Autodesk Inventor part; units mm, degrees
(part 2 of 2)
sketch "Эскиз30" plane through (0, 0, 0) normal (-1, 0, 0) x (0, 0, 1)
  circle A0 centre (-371.0468, 185.0848) radius 1.625 projected
  circle A1 centre (-103, 60) radius 2.1 projected
  circle A2 centre (-135.25, 60) radius 2.1 projected
  circle A3 centre (-173.9908, 56.343) radius 2.1 projected
  circle A4 centre (-50.8872, 165.0002) radius 2.1 projected
  circle A5 centre (-287, 56.343) radius 2.1 projected
  circle A6 centre (-319.1128, 165.0002) radius 2.1 projected
  arc A7 (-250, 372) -> (-253, 375) centre (-253, 372) ccw projected
  line L0 (-253, 375) -> (-377, 375) projected
  arc A8 (-377, 375) -> (-380, 372) centre (-377, 372) ccw projected
  line L1 (-380, 372) -> (-380, -2) projected
  arc A9 (-380, -2) -> (-377, -5) centre (-377, -2) ccw projected
  line L2 (-377, -5) -> (7, -5) projected
  arc A10 (7, -5) -> (10, -2) centre (7, -2) ccw projected
  line L3 (10, -2) -> (10, 372) projected
  arc A11 (10, 372) -> (7, 375) centre (7, 372) ccw projected
  line L4 (7, 375) -> (-117, 375) projected
  arc A12 (-117, 375) -> (-120, 372) centre (-117, 372) ccw projected
  line L5 (-120, 372) -> (-120, 323.5966) projected
  arc A13 (-123, 320.5966) -> (-120, 323.5966) centre (-123, 323.5966) ccw projected
  line L6 (-123, 320.5966) -> (-247, 320.5966) projected
  arc A14 (-250, 323.5966) -> (-247, 320.5966) centre (-247, 323.5966) ccw projected
  line L7 (-250, 323.5966) -> (-250, 372) projected
  arc A15 (-43, 338.848) -> (-40, 341.848) centre (-43, 341.848) ccw projected
  line L8 (-40, 341.848) -> (-40, 367) projected
  arc A16 (-37, 370) -> (-40, 367) centre (-37, 367) ccw projected
  line L9 (-37, 370) -> (-1, 370) projected
  arc A17 (2, 367) -> (-1, 370) centre (-1, 367) ccw projected
  line L10 (2, 367) -> (2, 269.848) projected
  arc A18 (-1, 266.848) -> (2, 269.848) centre (-1, 269.848) ccw projected
  line L11 (-1, 266.848) -> (-49, 266.848) projected
  arc A19 (-52, 269.848) -> (-49, 266.848) centre (-49, 269.848) ccw projected
  line L12 (-52, 269.848) -> (-52, 335.848) projected
  arc A20 (-49, 338.848) -> (-52, 335.848) centre (-49, 335.848) ccw projected
  line L13 (-49, 338.848) -> (-43, 338.848) projected
  arc A21 (-40, 28.152) -> (-43, 31.152) centre (-43, 28.152) ccw projected
  line L14 (-43, 31.152) -> (-49, 31.152) projected
  arc A22 (-52, 34.152) -> (-49, 31.152) centre (-49, 34.152) ccw projected
  line L15 (-52, 34.152) -> (-52, 100.152) projected
  arc A23 (-49, 103.152) -> (-52, 100.152) centre (-49, 100.152) ccw projected
  line L16 (-49, 103.152) -> (-43, 103.152) projected
  arc A24 (-43, 103.152) -> (-40, 106.152) centre (-43, 106.152) ccw projected
  line L17 (-40, 106.152) -> (-40, 160) projected
  arc A25 (-37, 163) -> (-40, 160) centre (-37, 160) ccw projected
  line L18 (-37, 163) -> (-1, 163) projected
  arc A26 (2, 160) -> (-1, 163) centre (-1, 160) ccw projected
  line L19 (2, 160) -> (2, 3) projected
  arc A27 (-1, 0) -> (2, 3) centre (-1, 3) ccw projected
  line L20 (-1, 0) -> (-37, 0) projected
  arc A28 (-40, 3) -> (-37, 0) centre (-37, 3) ccw projected
  line L21 (-40, 3) -> (-40, 28.152) projected
  line L22 (-165, 8) -> (-165, 44) projected
  arc A29 (-162, 47) -> (-165, 44) centre (-162, 44) ccw projected
  line L23 (-162, 47) -> (-96, 47) projected
  arc A30 (-93, 44) -> (-96, 47) centre (-96, 44) ccw projected
  line L24 (-93, 44) -> (-93, 8) projected
  arc A31 (-96, 5) -> (-93, 8) centre (-96, 8) ccw projected
  line L25 (-96, 5) -> (-162, 5) projected
  arc A32 (-165, 8) -> (-162, 5) centre (-162, 8) ccw projected
  circle A33 centre (-152.75, 251.9941) radius 2.1 projected
  circle A34 centre (-217.25, 118.0059) radius 2.1 projected
  circle A35 centre (-217.25, 57.0059) radius 2.1 projected
  circle A36 centre (-217.25, 251.9941) radius 2.1 projected
  circle A37 centre (-152.75, 312.9941) radius 2.1 projected
  circle A38 centre (-152.75, 118.0059) radius 2.1 projected
  circle A39 centre (-152.75, 57.0059) radius 2.1 projected
  circle A40 centre (-217.25, 312.9941) radius 2.1 projected
  circle A41 centre (-124.375, 193.0059) radius 2 projected
  circle A42 centre (-124.375, 129.0059) radius 2 projected
  line L26 (-98.825, 137.3849) -> (-98.825, 226.3849) projected
  arc A43 (-95.825, 229.3849) -> (-98.825, 226.3849) centre (-95.825, 226.3849) ccw projected
  line L27 (-95.825, 229.3849) -> (-87.825, 229.3849) projected
  arc A44 (-84.825, 226.3849) -> (-87.825, 229.3849) centre (-87.825, 226.3849) ccw projected
  line L28 (-84.825, 226.3849) -> (-84.825, 137.3849) projected
  arc A45 (-87.825, 134.3849) -> (-84.825, 137.3849) centre (-87.825, 137.3849) ccw projected
  line L29 (-87.825, 134.3849) -> (-95.825, 134.3849) projected
  arc A46 (-98.825, 137.3849) -> (-95.825, 134.3849) centre (-95.825, 137.3849) ccw projected
  line L30 (-358.5, 185.5001) -> (-358.5, 244.5001) projected
  arc A47 (-355.5, 247.5001) -> (-358.5, 244.5001) centre (-355.5, 244.5001) ccw projected
  line L31 (-355.5, 247.5001) -> (-335, 247.5001) projected
  arc A48 (-332, 244.5001) -> (-335, 247.5001) centre (-335, 244.5001) ccw projected
  line L32 (-332, 244.5001) -> (-332, 185.5001) projected
  arc A49 (-335, 182.5001) -> (-332, 185.5001) centre (-335, 185.5001) ccw projected
  line L33 (-335, 182.5001) -> (-355.5, 182.5001) projected
  arc A50 (-358.5, 185.5001) -> (-355.5, 182.5001) centre (-355.5, 185.5001) ccw projected
  line L34 (-35, 247.5001) -> (-14.5, 247.5001) projected
  arc A51 (-11.5, 244.5001) -> (-14.5, 247.5001) centre (-14.5, 244.5001) ccw projected
  line L35 (-11.5, 244.5001) -> (-11.5, 185.5001) projected
  arc A52 (-14.5, 182.5001) -> (-11.5, 185.5001) centre (-14.5, 185.5001) ccw projected
  line L36 (-14.5, 182.5001) -> (-35, 182.5001) projected
  arc A53 (-38, 185.5001) -> (-35, 182.5001) centre (-35, 185.5001) ccw projected
  line L37 (-38, 185.5001) -> (-38, 244.5001) projected
  arc A54 (-35, 247.5001) -> (-38, 244.5001) centre (-35, 244.5001) ccw projected
  arc A55 (-185, 192.7028) -> (-185, 193.309) centre (-183.175, 193.0059) ccw projected
  line L38 (-185, 192.7028) -> (-185, 193.309) projected
  circle A56 centre (-376, 368.9) radius 2.1 projected
  circle A57 centre (-299, 142) radius 1.625 projected
  circle A58 centre (-299, 2.0002) radius 1.625 projected
  circle A59 centre (-54, 368) radius 1.625 projected
  circle A60 centre (6, 1.1) radius 2.1 projected
  circle A61 centre (6, 368.9) radius 2.1 projected
  circle A62 centre (-54, 142) radius 1.625 projected
  circle A63 centre (1, 228) radius 1.625 projected
  circle A64 centre (-316, 2.0002) radius 1.625 projected
  circle A65 centre (-371, 228) radius 1.625 projected
  circle A66 centre (-299, 368) radius 1.625 projected
  circle A67 centre (-183.175, 129.0059) radius 1.85 projected
  circle A68 centre (-316, 228) radius 1.625 projected
  circle A69 centre (-316, 142) radius 1.625 projected
  circle A70 centre (-71, 228) radius 1.625 projected
  circle A71 centre (-71, 368) radius 1.625 projected
  circle A72 centre (-54, 2.0002) radius 1.625 projected
  circle A73 centre (-71, 2.0002) radius 1.625 projected
  circle A74 centre (-71, 142) radius 1.625 projected
  circle A75 centre (-54, 228) radius 1.625 projected
  circle A76 centre (-376, 1.1) radius 2.1 projected
  circle A77 centre (-299, 228) radius 1.625 projected
  circle A78 centre (-316, 368) radius 1.625 projected
  arc A79 (-330, 341.848) -> (-327, 338.848) centre (-327, 341.848) ccw projected
  line L39 (-327, 338.848) -> (-321, 338.848) projected
  arc A80 (-318, 335.848) -> (-321, 338.848) centre (-321, 335.848) ccw projected
  line L40 (-318, 335.848) -> (-318, 269.848) projected
  arc A81 (-321, 266.848) -> (-318, 269.848) centre (-321, 269.848) ccw projected
  line L41 (-321, 266.848) -> (-369, 266.848) projected
  arc A82 (-372, 269.848) -> (-369, 266.848) centre (-369, 269.848) ccw projected
  line L42 (-372, 269.848) -> (-372, 367) projected
  arc A83 (-369, 370) -> (-372, 367) centre (-369, 367) ccw projected
  line L43 (-369, 370) -> (-333, 370) projected
  arc A84 (-330, 367) -> (-333, 370) centre (-333, 367) ccw projected
  line L44 (-330, 367) -> (-330, 341.848) projected
  arc A85 (-327, 31.152) -> (-330, 28.152) centre (-327, 28.152) ccw projected
  line L45 (-330, 28.152) -> (-330, 3) projected
  arc A86 (-333, 0) -> (-330, 3) centre (-333, 3) ccw projected
  line L46 (-333, 0) -> (-369, 0) projected
  arc A87 (-372, 3) -> (-369, 0) centre (-369, 3) ccw projected
  line L47 (-372, 3) -> (-372, 160) projected
  arc A88 (-369, 163) -> (-372, 160) centre (-369, 160) ccw projected
  line L48 (-369, 163) -> (-333, 163) projected
  arc A89 (-330, 160) -> (-333, 163) centre (-333, 160) ccw projected
  line L49 (-330, 160) -> (-330, 106.152) projected
  arc A90 (-330, 106.152) -> (-327, 103.152) centre (-327, 106.152) ccw projected
  line L50 (-327, 103.152) -> (-321, 103.152) projected
  arc A91 (-318, 100.152) -> (-321, 103.152) centre (-321, 100.152) ccw projected
  line L51 (-318, 100.152) -> (-318, 34.152) projected
  arc A92 (-321, 31.152) -> (-318, 34.152) centre (-321, 34.152) ccw projected
  line L52 (-321, 31.152) -> (-327, 31.152) projected
  line L53 (-224.75, 65.0059) -> (-224.75, 110.0059) projected
  line L54 (-282, 51.343) -> (-282, 61.343) projected
  line L55 (-268.3252, 69.343) -> (-228.25, 69.343)
  line L56 (-226.25, 71.343) -> (-226.25, 99.9959)
  line L57 (-235.9248, 106.343) -> (-276, 106.343)
  line L58 (-278, 104.343) -> (-278, 75.6902)
  line L59 (-278, 69.343) -> (-226.25, 106.343)
  line L60 (-269.4885, 72.97) -> (-229.4132, 101.6228)
  line L61 (-274.8368, 74.0633) -> (-234.7615, 102.7161)
  arc A93 (-269.4885, 72.97) -> (-268.3252, 69.343) centre (-268.3252, 71.343) ccw
  arc A94 (-278, 75.6902) -> (-274.8368, 74.0633) centre (-276, 75.6902) ccw
  arc A95 (-234.7615, 102.7161) -> (-235.9248, 106.343) centre (-235.9248, 104.343) ccw
  arc A96 (-276, 106.343) -> (-278, 104.343) centre (-276, 104.343) ccw
  arc A97 (-228.25, 69.343) -> (-226.25, 71.343) centre (-228.25, 71.343) ccw
  arc A98 (-226.25, 99.9959) -> (-229.4132, 101.6228) centre (-228.25, 99.9959) ccw
  line L62 (-185, -235.3635) -> (-185, 601.2713)
  line L63 (-101.6748, 69.343) -> (-141.75, 69.343)
  line L64 (-143.75, 71.343) -> (-143.75, 99.9959)
  line L65 (-134.0752, 106.343) -> (-94, 106.343)
  line L66 (-92, 104.343) -> (-92, 75.6902)
  line L67 (-92, 69.343) -> (-143.75, 106.343)
  line L68 (-100.5115, 72.97) -> (-140.5868, 101.6228)
  line L69 (-95.1632, 74.0633) -> (-135.2385, 102.7161)
  arc A99 (-101.6748, 69.343) -> (-100.5115, 72.97) centre (-101.6748, 71.343) ccw
  arc A100 (-95.1632, 74.0633) -> (-92, 75.6902) centre (-94, 75.6902) ccw
  arc A101 (-134.0752, 106.343) -> (-135.2385, 102.7161) centre (-134.0752, 104.343) ccw
  arc A102 (-92, 104.343) -> (-94, 106.343) centre (-94, 104.343) ccw
  arc A103 (-143.75, 71.343) -> (-141.75, 69.343) centre (-141.75, 71.343) ccw
  arc A104 (-140.5868, 101.6228) -> (-143.75, 99.9959) centre (-141.75, 99.9959) ccw
  line L70 (-268.3252, 133.343) -> (-228.25, 133.343)
  line L71 (-226.25, 135.343) -> (-226.25, 163.9959)
  line L72 (-235.9248, 170.343) -> (-276, 170.343)
  line L73 (-278, 168.343) -> (-278, 139.6902)
  line L74 (-278, 133.343) -> (-226.25, 170.343)
  line L75 (-269.4885, 136.97) -> (-229.4132, 165.6228)
  line L76 (-274.8368, 138.0633) -> (-234.7615, 166.7161)
  arc A105 (-269.4885, 136.97) -> (-268.3252, 133.343) centre (-268.3252, 135.343) ccw
  arc A106 (-278, 139.6902) -> (-274.8368, 138.0633) centre (-276, 139.6902) ccw
  arc A107 (-234.7615, 166.7161) -> (-235.9248, 170.343) centre (-235.9248, 168.343) ccw
  arc A108 (-276, 170.343) -> (-278, 168.343) centre (-276, 168.343) ccw
  arc A109 (-228.25, 133.343) -> (-226.25, 135.343) centre (-228.25, 135.343) ccw
  arc A110 (-226.25, 163.9959) -> (-229.4132, 165.6228) centre (-228.25, 163.9959) ccw
  line L77 (-458.8698, 185) -> (88.8698, 185) projected
  line L78 (-268.3252, 300.657) -> (-228.25, 300.657)
  line L79 (-226.25, 298.657) -> (-226.25, 270.0041)
  line L80 (-235.9248, 263.657) -> (-276, 263.657)
  line L81 (-278, 265.657) -> (-278, 294.3098)
  line L82 (-278, 300.657) -> (-226.25, 263.657)
  line L83 (-269.4885, 297.03) -> (-229.4132, 268.3772)
  line L84 (-274.8368, 295.9367) -> (-234.7615, 267.2839)
  arc A111 (-268.3252, 300.657) -> (-269.4885, 297.03) centre (-268.3252, 298.657) ccw
  arc A112 (-274.8368, 295.9367) -> (-278, 294.3098) centre (-276, 294.3098) ccw
  arc A113 (-235.9248, 263.657) -> (-234.7615, 267.2839) centre (-235.9248, 265.657) ccw
  arc A114 (-278, 265.657) -> (-276, 263.657) centre (-276, 265.657) ccw
  arc A115 (-226.25, 298.657) -> (-228.25, 300.657) centre (-228.25, 298.657) ccw
  arc A116 (-229.4132, 268.3772) -> (-226.25, 270.0041) centre (-228.25, 270.0041) ccw
  line L85 (-134.0752, 263.657) -> (-94, 263.657)
  arc A117 (-94, 263.657) -> (-92, 265.657) centre (-94, 265.657) ccw
  arc A118 (-135.2385, 267.2839) -> (-134.0752, 263.657) centre (-134.0752, 265.657) ccw
  arc A119 (-143.75, 270.0041) -> (-140.5868, 268.3772) centre (-141.75, 270.0041) ccw
  line L86 (-92, 265.657) -> (-92, 294.3098)
  line L87 (-95.1632, 295.9367) -> (-135.2385, 267.2839)
  line L88 (-92, 300.657) -> (-143.75, 263.657)
  arc A120 (-100.5115, 297.03) -> (-101.6748, 300.657) centre (-101.6748, 298.657) ccw
  arc A121 (-92, 294.3098) -> (-95.1632, 295.9367) centre (-94, 294.3098) ccw
  line L89 (-101.6748, 300.657) -> (-141.75, 300.657)
  line L90 (-143.75, 298.657) -> (-143.75, 270.0041)
  arc A122 (-141.75, 300.657) -> (-143.75, 298.657) centre (-141.75, 298.657) ccw
  line L91 (-100.5115, 297.03) -> (-140.5868, 268.3772)
  arc A123 (-226.25, 230.3098) -> (-229.4132, 231.9367) centre (-228.25, 230.3098) ccw
  line L92 (-226.25, 201.657) -> (-226.25, 230.3098)
  arc A124 (-228.25, 199.657) -> (-226.25, 201.657) centre (-228.25, 201.657) ccw
  arc A125 (-278, 206.0041) -> (-274.8368, 204.3772) centre (-276, 206.0041) ccw
  arc A126 (-269.4885, 203.2839) -> (-268.3252, 199.657) centre (-268.3252, 201.657) ccw
  line L93 (-278, 234.657) -> (-278, 206.0041)
  arc A127 (-276, 236.657) -> (-278, 234.657) centre (-276, 234.657) ccw
  line L94 (-268.3252, 199.657) -> (-228.25, 199.657)
  line L95 (-235.9248, 236.657) -> (-276, 236.657)
  arc A128 (-234.7615, 233.03) -> (-235.9248, 236.657) centre (-235.9248, 234.657) ccw
  line L96 (-269.4885, 203.2839) -> (-229.4132, 231.9367)
  line L97 (-278, 199.657) -> (-226.25, 236.657)
  line L98 (-274.8368, 204.3772) -> (-234.7615, 233.03)
  arc A129 (-130.725, 234.2716) -> (-133.9769, 235.8314) centre (-132.725, 234.2716) ccw
  line L99 (-130.725, 206.0059) -> (-130.725, 234.2716)
  arc A130 (-138.3555, 237.4461) -> (-139.6074, 241.0059) centre (-139.6074, 239.0059) ccw
  line L100 (-167.9426, 204.0059) -> (-132.725, 204.0059)
  arc A131 (-169.1945, 207.5656) -> (-167.9426, 204.0059) centre (-167.9426, 206.0059) ccw
  line L101 (-169.1945, 207.5656) -> (-133.9769, 235.8314)
  line L102 (-176.825, 204.0059) -> (-130.725, 241.0059)
  line L103 (-173.5731, 209.1803) -> (-138.3555, 237.4461)
  line L104 (-139.6074, 241.0059) -> (-174.825, 241.0059)
  arc A132 (-176.825, 210.7401) -> (-173.5731, 209.1803) centre (-174.825, 210.7401) ccw
  line L105 (-176.825, 239.0059) -> (-176.825, 210.7401)
  arc A133 (-174.825, 241.0059) -> (-176.825, 239.0059) centre (-174.825, 239.0059) ccw
  arc A134 (-132.725, 204.0059) -> (-130.725, 206.0059) centre (-132.725, 206.0059) ccw
  line L106 (-130.725, 182.9338) -> (-130.725, 189.1279) projected
  point P0 (0, 0)
  point P1 (-145.25, 110.0059)
  point P2 (-255.9624, 106.343)
  point P3 (-224.75, 259.9941)
  point P4 (-145.25, 259.9941)
  point P5 (-255.9624, 263.657)
  point P6 (-226.25, 149.6695)
  point P7 (-176.825, 195.5059)
  dimension "d123" = 9
  dimension "d124" = 9
  dimension "d125" = 37
  dimension "d126" = 2
  dimension "d127" = 2
  dimension "d128" = 2
  dimension "d129" = 37
  dimension "d130" = 2
  dimension "d131" = 2
  dimension "d132" = 2
  dimension "d133" = 0
  dimension "d141" = 27
  dimension "d142" = 37
  dimension "d143" = 2
  dimension "d144" = 2
  dimension "d145" = 2
  dimension "d146" = 27
  dimension "d147" = 0
  dimension "d148" = 0
  dimension "d149" = 37
  dimension "d150" = 2
  dimension "d151" = 2
  dimension "d152" = 2
  dimension "d153" = 11
  dimension "d154" = 0
  dimension "d155" = 0
  constraints: 100 end point, 84 point on circle, 64 symmetric about line, 48 tangent, 42 centre point, 28 point on line, 20 equal radius, 16 parallel, 5 horizontal, 4 perpendicular, 2 midpoint, 1 vertical, 21 other
  measures "d123" distance from line of L58 A5.centre
  measures "d124" distance from line of A35.centre L56
  measures "d125" distance between parallel lines of L57 L55
  measures "d126" distance between parallel lines of L59 L60
  measures "d127" distance between parallel lines of L59 L61
  measures "d128" radius of A93
  measures "d129" distance between parallel lines of L72 L70
  measures "d130" distance between parallel lines of L74 L75
  measures "d131" distance between parallel lines of L74 L76
  measures "d132" radius of A105
  measures "d133" distance between parallel lines of L58 L73
  measures "d141" distance between parallel lines of L57 L70
  measures "d142" distance between parallel lines of L95 L94
  measures "d143" distance between parallel lines of L97 L96
  measures "d144" distance between parallel lines of L97 L98
  measures "d145" radius of A126
  measures "d146" distance between parallel lines of L95 L80
  measures "d147" distance between parallel lines of L73 L93
  measures "d148" distance from line of point (-226.25, 149.669) L92
  measures "d149" distance between parallel lines of L104 L100
  measures "d150" distance between parallel lines of L102 L101
  measures "d151" distance between parallel lines of L102 L103
  measures "d152" radius of A131
  measures "d153" distance from line of A55.centre L100
  measures "d154" distance from line of point (-176.825, 195.506) L105
  measures "d155" distance between parallel lines of L106 L99
extrude "Выдавливание27" cut sketch "Эскиз30" against normal blind 10 contours A93 L60 A98 L56 A97 L55 | A95 L61 A94 L58 A96 L57 | L63 A103 L64 A104 L68 A99 | L65 A102 L66 A100 L69 A101 | A105 L75 A110 L71 A109 L70 | A107 L76 A106 L73 A108 L72 | L78 A115 L79 A116 L83 A111 | L80 A114 L81 A112 L84 A113 | A118 L87 A121 L86 A117 L85 | L90 A122 L89 A120 L91 A119 | L92 A124 L94 A126 L96 A123 | L93 A127 L95 A128 L98 A125 | L99 A134 L100 A131 L101 A129 | L103 A132 L105 A133 L104 A130
sketch "Эскиз31" plane through (1.5, 0, 0) normal (1, 0, 0) x (0, 0, -1)
  point P0 (0, 0)
equation "\"d99\" = d97"
